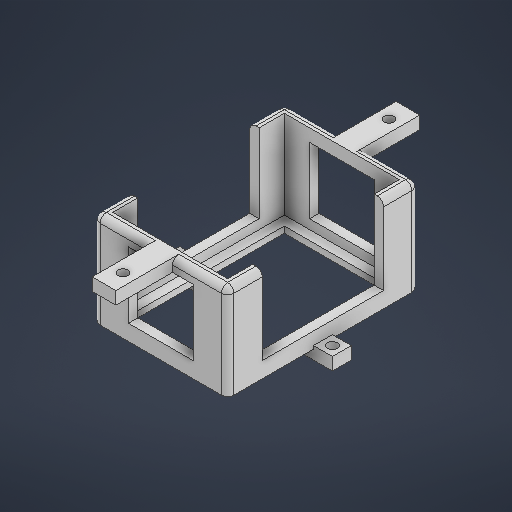
# Autodesk Inventor part: mocowanie-controller
Saved by Autodesk Inventor 2026.2 (Build 302298010, 298A)
## iProperties
Created: 2026-04-19
Part Number: mocowanie-controller
Material: Ogólny
Document SubType Name: Modeling
Designer: macie
Density: 1 g/cm^3
Appearance: Domyślna
Author: macie
Autodesk Inventor part; units mm, degrees
ref_plane "YZ Plane" through (0, 0, 0) normal (1, 0, 0) x (0, 1, 0)
ref_plane "XZ Plane" through (0, 0, 0) normal (0, 1, 0) x (-1, 0, 0)
ref_plane "XY Plane" through (0, 0, 0) normal (0, 0, 1) x (1, 0, 0)
sketch "Szkic1" plane through (0, 0, 0) normal (0, 1, 0) x (-1, 0, 0)
  line L0 (18.25, 27.25) -> (-18.25, 27.25)
  line L1 (-18.25, 27.25) -> (-18.25, -27.25)
  line L2 (-18.25, -27.25) -> (18.25, -27.25)
  line L3 (18.25, -27.25) -> (18.25, 27.25)
  line L4 (18.25, 27.25) -> (-18.25, -27.25) construction
  line L5 (-18.25, 27.25) -> (18.25, -27.25) construction
  line L6 (21.25, 30.25) -> (-21.25, 30.25)
  line L7 (-21.25, 30.25) -> (-21.25, -30.25)
  line L8 (-21.25, -30.25) -> (21.25, -30.25)
  line L9 (21.25, -30.25) -> (21.25, 30.25)
  line L10 (21.25, 30.25) -> (-21.25, -30.25) construction
  line L11 (-21.25, 30.25) -> (21.25, -30.25) construction
  line L12 (15.25, 24.25) -> (-15.25, 24.25)
  line L13 (-15.25, 24.25) -> (-15.25, -24.25)
  line L14 (-15.25, -24.25) -> (15.25, -24.25)
  line L15 (15.25, -24.25) -> (15.25, 24.25)
  line L16 (15.25, 24.25) -> (-15.25, -24.25) construction
  line L17 (-15.25, 24.25) -> (15.25, -24.25) construction
  point P0 (0, 0)
  dimension "d0" = 54.5
  dimension "d1" = 36.5
  dimension "d2" = 42.5
  dimension "d3" = 60.5
  dimension "d4" = 48.5
  dimension "d5" = 30.5
  constraints: 36 end point, 6 midpoint, 6 parallel, 3 horizontal, 3 perpendicular
  measures "d0" distance between parallel lines of L2 L0
  measures "d1" distance between parallel lines of L1 L3
  measures "d2" distance between parallel lines of L7 L9
  measures "d3" distance between parallel lines of L8 L6
  measures "d4" distance between parallel lines of L14 L12
  measures "d5" distance between parallel lines of L13 L15
extrude "Wyciągnięcie proste1" add sketch "Szkic1" along normal blind 5 contours L9 L8 L7 L6
extrude "Wyciągnięcie proste2" add sketch "Szkic1" along normal blind 2 contours L3 L2 L1 L0
sketch "Szkic2" plane through (0, 5, 0) normal (0, 1, 0) x (1, 0, 0)
  line L0 (-21.25, -30.25) -> (21.25, -30.25) projected
  line L1 (-18.25, -27.25) -> (-18.25, 27.25) projected
  line L2 (-21.25, -30.25) -> (-18.25, -30.25)
  line L3 (-18.25, -30.25) -> (-18.25, -19.25)
  line L4 (-18.25, -19.25) -> (-21.25, -19.25)
  line L5 (-21.25, -19.25) -> (-21.25, -30.25)
  line L6 (-18.25, -27.25) -> (-10.25, -27.25)
  line L7 (-10.25, -27.25) -> (-10.25, -30.25)
  line L8 (-10.25, -30.25) -> (-18.25, -30.25)
  line L9 (-18.25, -30.25) -> (-18.25, -27.25)
  line L10 (18.25, 30.25) -> (18.25, 19.25)
  line L11 (21.25, 30.25) -> (18.25, 30.25)
  line L12 (21.25, 19.25) -> (21.25, 30.25)
  line L13 (18.25, 19.25) -> (21.25, 19.25)
  line L14 (18.25, 27.25) -> (10.25, 27.25)
  line L15 (10.25, 30.25) -> (18.25, 30.25)
  line L16 (10.25, 27.25) -> (10.25, 30.25)
  line L17 (21.25, -30.25) -> (21.25, 30.25) projected
  line L18 (18.25, 27.25) -> (18.25, -27.25) projected
  line L19 (21.25, -30.25) -> (18.25, -30.25)
  line L20 (18.25, -30.25) -> (18.25, -19.25)
  line L21 (18.25, -19.25) -> (21.25, -19.25)
  line L22 (21.25, -19.25) -> (21.25, -30.25)
  line L23 (18.25, -27.25) -> (10.25, -27.25)
  line L24 (10.25, -27.25) -> (10.25, -30.25)
  line L25 (10.25, -30.25) -> (18.25, -30.25)
  line L26 (18.25, -30.25) -> (18.25, -27.25)
  line L27 (-10.25, 27.25) -> (-10.25, 30.25)
  line L28 (-10.25, 30.25) -> (-18.25, 30.25)
  line L29 (-21.25, 30.25) -> (-18.25, 30.25)
  line L30 (-21.25, 19.25) -> (-21.25, 30.25)
  line L31 (-18.25, 19.25) -> (-21.25, 19.25)
  line L32 (-18.25, 30.25) -> (-18.25, 19.25)
  line L33 (-18.25, 27.25) -> (-10.25, 27.25)
  point P0 (0, 0)
  point P1 (-19.75, -30.25)
  point P2 (-19.75, -19.25)
  point P3 (19.75, 30.25)
  point P4 (19.75, 19.25)
  point P5 (18.25, 27.25)
  point P6 (-18.25, 27.25)
  dimension "d10" = 11
  dimension "d11" = 8
  dimension "d14" = 360
  dimension "d16" = 8
  dimension "d17" = 11
  dimension "d20" = 360
  constraints: 60 end point, 8 parallel, 5 point on line, 4 horizontal, 4 perpendicular, 2 midpoint, 66 other
  measures "d10" distance of point (-19.75, -30.25) point (-19.75, -19.25)
  measures "d11" distance between parallel lines of L7 L3
  measures "d16" distance between parallel lines of L26 L24
  measures "d17" distance between parallel lines of L0 L21
extrude "Wyciągnięcie proste3" add sketch "Szkic2" along normal blind 25 contours L5 L4 L1 L3 L0 | L3 L6 L7 L0 | L24 L23 L20 L0 | L20 L18 L21 L17 L0 | L13 L10 L11 L12 | L14 L16 L15 L10 | L31 L30 L29 L32 L1 | L32 L28 L27 L33
sketch "Szkic3" plane through (-10.25, 5, 30.25) normal (1, 0, 0) x (0, 0, -1)
  line L0 (0, 0) -> (0, 25) projected
  line L1 (3, 0) -> (3, 25) projected
  line L2 (0, 25) -> (3, 25)
  line L3 (3, 25) -> (3, 21)
  line L4 (3, 21) -> (0, 21)
  line L5 (0, 21) -> (0, 25)
  line L6 (57.5, 0) -> (57.5, 25) projected
  line L7 (60.5, -5) -> (60.5, 25) projected
  line L8 (57.5, 25) -> (60.5, 25)
  line L9 (60.5, 25) -> (60.5, 21)
  line L10 (60.5, 21) -> (57.5, 21)
  line L11 (57.5, 21) -> (57.5, 25)
  point P0 (30.25, -5)
  point P1 (0, 21)
  dimension "d24" = 4
  dimension "d27" = 4
  constraints: 16 end point, 4 parallel, 2 horizontal, 2 perpendicular, 2 point on line
  measures "d24" distance between parallel lines of L4 L2
  measures "d27" distance between parallel lines of L10 L8
extrude "Wyciągnięcie proste4" add sketch "Szkic3" along normal blind 21
sketch "Szkic4" plane through (-21.25, 0, 30.25) normal (0, 0, 1) x (1, 0, 0)
  line L0 (3, 30) -> (39.5, 30) projected
  line L1 (11, 26) -> (31.5, 26) projected
  line L2 (17.4935, 30) -> (25.0065, 30)
  line L3 (25.0065, 30) -> (25.0065, 26)
  line L4 (25.0065, 26) -> (17.4935, 26)
  line L5 (17.4935, 26) -> (17.4935, 30)
  line L6 (0, 0) -> (0, 30) projected
  point P0 (21.25, 0)
  dimension "d28" = 7.513
  dimension "d29" = 17.4935
  constraints: 8 end point, 2 parallel, 2 point on line, 1 horizontal, 1 perpendicular
  measures "d28" distance between parallel lines of L3 L5
  measures "d29" distance between parallel lines of L6 L5
extrude "Wyciągnięcie proste5" add sketch "Szkic4" along normal blind 18
mirror "Odbij1" about plane through (0, 0, 0) normal (0, 0, 1) of "Wyciągnięcie proste5"
sketch "Szkic5" plane through (0, 30, 0) normal (0, 1, 0) x (1, 0, 0)
  line L0 (3.7565, -48.25) -> (-3.7565, -48.25) projected
  line L1 (3.7565, -30.25) -> (3.7565, -48.25) projected
  point P0 (0, 0)
  point P1 (0, -42.25)
  dimension "d32" = 6
  dimension "d33" = 3.7565
  measures "d32" distance from line of point (0, -42.25) L0
  measures "d33" distance from line of L1 point (0, -42.25)
hole "Otwór1" at (0, 30, 42.25) direction (0, -1, 0) diameter 3.2 end through all
mirror "Odbij2" about plane through (0, 0, 0) normal (0, 0, 1) of "Otwór1"
fillet "Zaokrąglenie1" radius 2 12 edges at (12.5032, 30, 30.25) (21.25, 30, 24.75) (21.25, 15, 30.25) (21.25, 30, -24.75) (21.25, 15, -30.25) (12.5032, 30, -30.25) (-21.25, 30, 24.75) (-12.5033, 30, 30.25) (-21.25, 15, 30.25) (-21.25, 15, -30.25) (-21.25, 30, -24.75) (-12.5032, 30, -30.25)
sketch "Szkic6" plane through (0, 0, 0) normal (0, -1, 0) x (1, 0, 0)
  line L0 (-21.25, -28.25) -> (-21.25, 28.25) projected
  line L1 (-15.25, 24.25) -> (-15.25, -24.25) projected
  line L2 (-21.25, 3) -> (-15.25, 3)
  line L3 (-15.25, 3) -> (-15.25, -3)
  line L4 (-15.25, -3) -> (-21.25, -3)
  line L5 (-21.25, -3) -> (-21.25, 3)
  line L6 (21.25, -3) -> (15.25, -3)
  line L7 (21.25, 3) -> (21.25, -3)
  line L8 (15.25, -3) -> (15.25, 3)
  line L9 (15.25, 3) -> (21.25, 3)
  point P0 (0, 0)
  point P1 (-21.25, 0)
  dimension "d42" = 6
  dimension "d43" = 3
  dimension "d46" = 360
  constraints: 16 end point, 2 parallel, 2 point on line, 1 horizontal, 1 midpoint, 1 perpendicular, 17 other
  measures "d42" distance between parallel lines of L4 L2
  measures "d43" distance from line of point (-21.25, 0) L2
extrude "Wyciągnięcie proste6" add sketch "Szkic6" along normal blind 3
sketch "Szkic7" plane through (-21.25, 5, -19.25) normal (-1, 0, 0) x (0, 0, 1)
  line L0 (22.25, -8) -> (16.25, -8) projected
  line L1 (16.25, -8) -> (22.25, -8)
  line L2 (22.25, -8) -> (22.25, -4)
  line L3 (22.25, -4) -> (16.25, -4)
  line L4 (16.25, -4) -> (16.25, -8)
  line L5 (22.25, -6) -> (16.25, -6)
  line L6 (16.25, -6) -> (16.25, -8)
  line L7 (16.25, -8) -> (22.25, -8)
  line L8 (22.25, -8) -> (22.25, -6)
  point P0 (19.25, -5)
  point P1 (19.25, -4)
  point P2 (19.25, -6)
  point P3 (22.25, -8)
  dimension "d50" = 3
  dimension "d52" = 1
  dimension "d53" = 2
  dimension "d54" = 0
  constraints: 16 end point, 4 parallel, 3 midpoint, 2 horizontal, 2 perpendicular, 1 point on line
  measures "d50" distance from line of point (19.25, -5) L2
  measures "d52" distance of point (19.25, -4) point (19.25, -5)
  measures "d53" distance from line of point (19.25, -6) L7
  measures "d54" distance between parallel lines of L0 L7
extrude "Wyciągnięcie proste7" add sketch "Szkic7" along normal blind 6
mirror "Odbij3" about plane through (0, 0, 0) normal (1, 0, 0) of "Wyciągnięcie proste7"
sketch "Szkic8" plane through (-21.25, 1, 3) normal (0, 1, 0) x (1, 0, 0)
  line L0 (-6, 0) -> (-6, 6) projected
  line L1 (0, 0) -> (-6, 0) projected
  line L2 (42.5, -16.25) -> (42.5, 22.25) projected
  line L3 (42.5, 6) -> (48.5, 6) projected
  point P0 (21.25, 3)
  point P1 (-3, 3)
  point P2 (-6, 3)
  point P3 (-3, 0)
  point P4 (45.5, 3)
  dimension "d57" = 3
  dimension "d58" = 3
  dimension "d59" = 3
  dimension "d60" = 3
  constraints: 2 midpoint
  measures "d57" distance of point (-6, 3) point (-3, 3)
  measures "d58" distance of point (-3, 0) point (-3, 3)
  measures "d59" distance from line of L2 point (45.5, 3)
  measures "d60" distance from line of L3 point (45.5, 3)
hole "Otwór2" at (-24.25, 1, 0) at (24.25, 1, 0) direction (0, -1, 0) diameter 3.2 end through all
equation "\"d59\" = d57"
equation "\"d60\" = d58"
